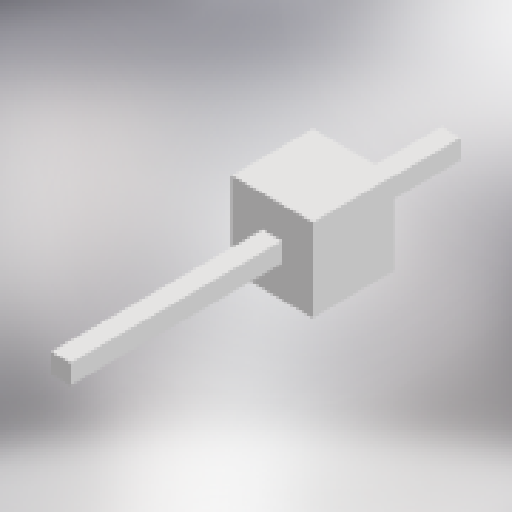
# Autodesk Inventor part: Header D1
Saved by Autodesk Inventor 2024 (Build 280153000, 153)
## iProperties
Created: 2024-10-31
Part Number: Header D1
Material: Generic
Document SubType Name: Modeling
Designer: Tejas
Mass: 0.019295 g
Surface Area: 0.607 cm^2
Volume: 0.019295 cm^3
Density: 1 g/cm^3
Appearance: Default
Author: Tejas
Autodesk Inventor part; units mm, degrees
ref_plane "YZ Plane" through (0, 0, 0) normal (1, 0, 0) x (0, 1, 0)
ref_plane "XZ Plane" through (0, 0, 0) normal (0, 1, 0) x (-1, 0, 0)
ref_plane "XY Plane" through (0, 0, 0) normal (0, 0, 1) x (1, 0, 0)
sketch "Sketch2" plane through (0, 0, 0) normal (0, 0, 1) x (1, 0, 0)
  line L0 (-0.3, 0.3) -> (0.3, 0.3)
  line L1 (0.3, 0.3) -> (0.3, -0.3)
  line L2 (0.3, -0.3) -> (-0.3, -0.3)
  line L3 (-0.3, -0.3) -> (-0.3, 0.3)
  line L4 (-0.3, 0.3) -> (0.3, -0.3) construction
  line L5 (0.3, 0.3) -> (-0.3, -0.3) construction
  point P0 (0, 0)
  dimension "d2" = 0.6
  dimension "d3" = 0.6
  constraints: 12 end point, 2 midpoint, 2 parallel, 1 horizontal, 1 perpendicular
  measures "d2" distance of L1.end L2.end
  measures "d3" distance of L0.end L1.end
extrude "Extrusion1" add sketch "Sketch2" along normal blind 10 and the other way blind 2
sketch "Sketch3" plane through (0, 0, -2) normal (0, 0, -1) x (-1, 0, 0)
  line L0 (-0.3, -0.3) -> (0.3, -0.3) projected
  line L1 (0.3, -0.3) -> (0.3, 0.3) projected
  line L2 (0.3, 0.3) -> (-0.3, 0.3) projected
  line L3 (-0.3, 0.3) -> (-0.3, -0.3) projected
  line L4 (-1.25, 1.27) -> (1.25, 1.27)
  line L5 (1.25, 1.27) -> (1.25, -1.27)
  line L6 (1.25, -1.27) -> (-1.25, -1.27)
  line L7 (-1.25, -1.27) -> (-1.25, 1.27)
  line L8 (-1.25, 1.27) -> (1.25, -1.27) construction
  line L9 (1.25, 1.27) -> (-1.25, -1.27) construction
  point P0 (0, 0)
  dimension "d8" = 2.54
  dimension "d9" = 2.5
  constraints: 12 end point, 2 midpoint, 2 parallel, 1 horizontal, 1 perpendicular
  measures "d8" distance of L4.end L5.end
  measures "d9" distance of L5.end L6.end
ref_plane "Work Plane1" through (0, 0, 1) normal (0, 0, -1) x (-1, 0, 0)
extrude "Extrusion2" add sketch "Sketch3" against normal blind 2.5 from surface at -3
body "Solid1"
